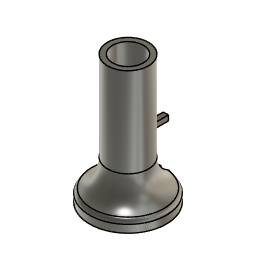
Pawn bottom part (Autodesk Fusion 360 design; units mm, degrees)
Autodesk Fusion 360 part; units mm, degrees
sketch "Sketch1" plane through (0, 0, 0) normal (0, 0, 1) x (1, 0, 0)
  circle A0 centre (0, 0) radius 15
  constraint coincident A0.centre origin
extrude "Extrude1" add sketch "Sketch1" along normal blind 5 makes body 1
sketch "Sketch2" plane through (0, 0, 5) normal (0, 0, 1) x (-1, 0, 0)
  circle A0 centre (0, 0) radius 15
  circle A1 centre (0, 0) radius 8
  constraint coincident A0.centre A1.centre
extrude "Extrude2" add sketch "Sketch2" along normal blind 45 contours A1 bodies 1
fillet "Fillet1" radius 2 1 edges at (-13.9849, -5.4242, 5) on bodies 1
fillet "Fillet2" radius 12 1 edges at (7.4586, -2.8929, 5) on bodies 1
shell "Shell1" thickness 2 removed faces 1 at (-1.8969, -2.8445, 50) on bodies 1
sketch "Sketch3" plane through (0, 0, 0) normal (0, 0, 1) x (1, 0, 0)
  circle A0 centre (40, 0) radius 2
  circle A1 centre (40, 0) radius 6
  constraint concentric A0 A1
extrude "Extrude3" add sketch "Sketch3" along normal blind 2 separate body makes body 2
move_body "Move1" bodies 2 to x (1, 0, 0) y (0, 1, 0) z (0, 0, 1) at (0, 0, 27)
move_body "Move2" bodies 2 to x (1, 0, 0) y (0, 1, 0) z (0, 0, 1) at (-40, 0, 0)
combine "Combine1" operation add target body 2 tool bodies 1
sketch "Sketch4" plane through (0, 0, 0) normal (0, 1, 0) x (1, 0, 0)
  line L0 (0, -2) -> (1.75, -2)
  line L1 (1.75, -2) -> (1.75, -24)
  line L2 (1.75, -24) -> (0, -24)
  line L3 (0, -2) -> (-1.75, -2)
  line L4 (-1.75, -2) -> (-1.75, -24)
  line L5 (-1.75, -24) -> (0, -24)
  dimension "d12" = 1.75
  dimension "d13" = 22
  dimension "d14" = 22
  constraint horizontal L0
  constraint vertical L1
  constraint horizontal L2
  constraint horizontal L3
  constraint vertical L4
  constraint horizontal L5
  measures "d12" distance of L0.start L0.end
  measures "d13" distance of L0.start L2.end
  measures "d14" distance of L0.start L2.end
extrude "Extrude4" cut sketch "Sketch4" along normal blind 15 bodies 2
sketch "Sketch5" plane through (0, 0, 0) normal (1, 0, 0) x (0, 1, 0)
  line L0 (35, 2) -> (35, 22.5)
  line L1 (35, 22.5) -> (42, 22.5)
  line L2 (42, 22.5) -> (42, 20.5)
  line L3 (42, 20.5) -> (35, 20.5)
  line L4 (35, 20.5) -> (35, 22.5)
  line L5 (35, 22.5) -> (33, 22.5)
  line L6 (33, 22.5) -> (33, 2)
  line L7 (33, 2) -> (35, 2)
  line L8 (33, 22.5) -> (33, 19)
  line L9 (33, 19) -> (29.5, 19)
  line L10 (33, 22.5) -> (29.5, 19)
  dimension "d17" = 20.5
  dimension "d18" = 7
  dimension "d19" = 2
  dimension "d20" = 3.5
  dimension "d21" = 3.5
  constraint vertical L0
  constraint horizontal L1
  constraint vertical L2
  constraint horizontal L3
  constraint vertical L4
  constraint perpendicular L0 L5
  constraint perpendicular L5 L6
  constraint perpendicular L0 L7
  constraint perpendicular L5 L8
  constraint perpendicular L6 L9
  measures "d17" distance of L0.start L0.end
  measures "d18" distance of L0.end L1.end
  measures "d19" distance of L0.end L3.end
  measures "d20" distance of L5.end L8.end
  measures "d21" distance of L8.end L9.end
extrude "Extrude5" add sketch "Sketch5" along normal blind 2 separate body makes body 3
move_body "Move3" bodies 3 to x (1, 0, 0) y (0, 1, 0) z (0, 0, 1) at (-1, -27.2, 0)
combine "Combine2" operation add target body 3 tool bodies 2
